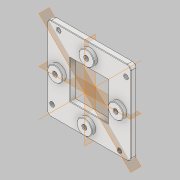
# Autodesk Inventor part: BaseTop
Saved by Autodesk Inventor 2019.2 (Build 232265000, 265)
## iProperties
Created: 2019-01-12
Part Number: BaseTop
Material: ABS-Kunststoff
Document SubType Name: Modeling
Designer: Lion
Density: 1.06 g/cm^3
Appearance: Weiß
Mass: 6.25719 g
Surface Area: 43.195 cm^2
Volume: 5.90301 cm^3
Author: Lion
## iProperties of the stored document BaseTop_3D-Druck.ipt
Created: 2019-04-11
Part Number: BaseTop_3D-Druck
Material: Generisch
Document SubType Name: Modeling
Designer: Lion
Density: 1 g/cm^3
Appearance: Vorgabe
Author: Lion
Autodesk Inventor part; units mm, degrees
ref_plane "YZ Plane" through (0, 0, 0) normal (1, 0, 0) x (0, 1, 0)
ref_plane "XZ Plane" through (0, 0, 0) normal (0, 1, 0) x (-1, 0, 0)
ref_plane "XY Plane" through (0, 0, 0) normal (0, 0, 1) x (1, 0, 0)
sketch "Skizze2" plane through (0, 0, 0) normal (0, 0, 1) x (1, 0, 0)
  line L0 (-16, -6) -> (16, -6)
  line L1 (16, -6) -> (16, 6)
  line L2 (16, 6) -> (-16, 6)
  line L3 (-16, 6) -> (-16, -6)
  line L4 (-16, -6) -> (16, 6) construction
  line L5 (16, -6) -> (-16, 6) construction
  line L6 (-11, 6) -> (3, 6)
  line L7 (3, 6) -> (3, -6)
  line L8 (3, -6) -> (-11, -6)
  line L9 (-11, -6) -> (-11, 6)
  circle A0 centre (-13.5, 0) radius 1
  line L10 (-11, -6) -> (-16, 6) construction
  line L11 (-16, -6) -> (-11, 6) construction
  line L12 (0, 6) -> (0, -6) construction
  circle A1 centre (13.5, 0) radius 1
  line L13 (-16, -21) -> (-28, -26) construction
  line L14 (-28, -7) -> (-16, -7)
  line L15 (-28, -10) -> (-16, -10) construction
  line L16 (-16, -26) -> (-16, 6)
  line L17 (-28, 6) -> (-28, -26)
  line L18 (-16, -26) -> (-28, 6) construction
  line L19 (-16, 6) -> (-28, -26) construction
  line L20 (-16, -21) -> (-28, -21)
  line L21 (-16, -7) -> (-16, -21)
  line L22 (-16, -26) -> (-28, -21) construction
  line L23 (-28, -26) -> (-16, -26)
  circle A2 centre (-22, -23.5) radius 1
  line L24 (-28, -21) -> (-28, -7)
  circle A3 centre (-22, 3.5) radius 1
  line L25 (-16, 6) -> (-28, 6)
  line L26 (-15, -38) -> (-15, -26)
  circle A4 centre (-25.5, -32) radius 1
  line L27 (-28, -26) -> (-28, -38)
  line L28 (-12, -38) -> (-12, -26) construction
  line L29 (4, -26) -> (-28, -26)
  line L30 (-28, -26) -> (4, -38) construction
  line L31 (4, -26) -> (-28, -38) construction
  line L32 (-28, -38) -> (4, -38)
  line L33 (-15, -26) -> (-1, -26)
  line L34 (-1, -38) -> (-15, -38)
  line L35 (-1, -26) -> (-1, -38)
  circle A5 centre (1.5, -32) radius 1
  line L36 (4, -26) -> (-1, -38) construction
  line L37 (-1, -26) -> (4, -38) construction
  line L38 (4, -38) -> (4, -26)
  line L39 (16, -25) -> (4, -25)
  circle A6 centre (10, -35.5) radius 1
  line L40 (4, -38) -> (16, -38)
  line L41 (16, -22) -> (4, -22) construction
  line L42 (4, -6) -> (4, -38)
  line L43 (4, -38) -> (16, -6) construction
  line L44 (4, -6) -> (16, -38) construction
  line L45 (16, -38) -> (16, -6)
  line L46 (4, -25) -> (4, -11)
  line L47 (16, -11) -> (16, -25)
  line L48 (4, -11) -> (16, -11)
  circle A7 centre (10, -8.5) radius 1
  line L49 (4, -6) -> (16, -11) construction
  line L50 (4, -11) -> (16, -6) construction
  line L51 (16, -6) -> (4, -6)
  line L52 (-16, -26) -> (4, -6) construction
  line L53 (4, -26) -> (-16, -6) construction
  line L54 (1, -23) -> (-13, -23)
  line L55 (-13, -23) -> (-13, -9)
  line L56 (-13, -9) -> (1, -9)
  line L57 (1, -9) -> (1, -23)
  line L58 (1, -23) -> (-13, -9) construction
  line L59 (-13, -23) -> (1, -9) construction
  line L60 (4, -25) -> (16, -25)
  line L61 (16, -25) -> (16, -38)
  line L62 (16, -38) -> (4, -38)
  line L63 (4, -38) -> (4, -25)
  point P0 (0, 0)
  point P1 (-13.5, 0)
  point P2 (-22, -10)
  point P3 (-12, -32)
  point P4 (10, -22)
  point P5 (-6, -16)
sketch "Skizze3" plane through (0, 0, 0) normal (0, 0, 1) x (1, 0, 0)
  circle A0 centre (-25.5, -32) radius 1 construction
  circle A1 centre (10, -35.5) radius 1 construction
  circle A2 centre (-22, 3.5) radius 1 construction
  circle A3 centre (13.5, 0) radius 1 construction
  line L0 (-28, 6) -> (16, 6)
  line L1 (16, 6) -> (16, -38)
  line L2 (16, -38) -> (-28, -38)
  line L3 (-28, -38) -> (-28, 6)
  circle A4 centre (-22, 3.5) radius 1
  circle A5 centre (13.5, 0) radius 1
  circle A6 centre (10, -35.5) radius 1
  circle A7 centre (-25.5, -32) radius 1
  line L4 (-16, -6) -> (4, -6)
  line L5 (4, -6) -> (4, -26)
  line L6 (4, -26) -> (-16, -26)
  line L7 (-16, -26) -> (-16, -6)
  line L8 (-11, -6) -> (-11, 6) construction
  line L9 (4, -11) -> (16, -11) construction
  line L10 (-1, -26) -> (-1, -38) construction
  line L11 (-16, -21) -> (-28, -21) construction
  circle A8 centre (-22, -15.5) radius 1.05
  line L12 (-22, -10) -> (-22, -23.5) construction
  line L13 (-12, -32) -> (1.5, -32) construction
  line L14 (10, -22) -> (10, -8.5) construction
  line L15 (-13.5, 0) -> (0, 0) construction
  circle A9 centre (10, -16.5) radius 1.05
  circle A10 centre (-5.5, 0) radius 1.05
  circle A11 centre (-6.5, -32) radius 1.05
  point P0 (-28, -38)
  point P1 (16, 6)
  point P2 (-16, -26)
  point P3 (4, -6)
  dimension "leghole_top_d" = 2.1
  dimension "d2" = 5.5
  dimension "d3" = 2.1
  dimension "d4" = 2.1
  dimension "d5" = 2.1
  dimension "d6" = 5.5
  dimension "d7" = 5.5
  dimension "d8" = 5.5
  constraints: 24 end point, 8 centre point, 4 coincident, 4 concentric, 4 horizontal, 4 parallel, 4 point on line, 2 perpendicular, 2 vertical
  measures "leghole_top_d" diameter of A8
  measures "d2" distance from line of L11 A8.centre
  measures "d3" diameter of A9
  measures "d4" diameter of A10
  measures "d5" diameter of A11
  measures "d6" distance from line of A11.centre L10
  measures "d7" distance from line of L9 A9.centre
  measures "d8" distance from line of L8 A10.centre
extrude "Extrusion1" add sketch "Skizze3" along normal blind 3
sketch "Skizze6" plane through (0, 0, 3) normal (0, 0, 1) x (1, 0, 0)
  circle A0 centre (-5.5, 0) radius 1.05 projected
  circle A1 centre (10, -16.5) radius 1.05 projected
  circle A2 centre (-22, -15.5) radius 1.05 projected
  circle A3 centre (-6.5, -32) radius 1.05 projected
  circle A4 centre (-5.5, 0) radius 4
  circle A5 centre (10, -16.5) radius 4
  circle A6 centre (-6.5, -32) radius 1.05 projected
  circle A7 centre (-6.5, -32) radius 4
  circle A8 centre (-22, -15.5) radius 4
  point P0 (0, 0)
  dimension "d18" = 8
  constraints: 4 centre point, 4 coincident, 3 equal radius
  measures "d18" diameter of A4
extrude "Extrusion3" add sketch "Skizze6" along normal blind 2
fillet "Rundung1" radius 2 4 edges at (-28, -38, 1.5) (16, -38, 1.5) (16, 6, 1.5) (-28, 6, 1.5)
ref_plane "Arbeitsebene1" through (-16, -6, 0) normal (0.7071068, 0.7071068, 0) x (0, 0, 1)
ref_plane "Arbeitsebene2" through (-16, -26, 0) normal (-0.7071068, 0.7071068, 0) x (0, 0, 1)
ref_plane "Arbeitsebene3" through (-6, -36, 0) normal (1, 0, 0) x (0, 0, -1)
ref_plane "Arbeitsebene4" through (-26, -16, 0) normal (0, 1, 0) x (1, 0, 0)
fillet "Rundung2" radius 0.25 44 edges at (-6, 6, 0) (-6, 6, 3) (-27.4142, 5.4142, 0) (15.4142, 5.4142, 0) (-28, -16, 0) (16, -16, 0) (-27.4142, -37.4142, 0) (15.4142, -37.4142, 0) (-6, -38, 0) (-26.5, -32, 0) (-7.55, -32, 0) (9, -35.5, 0) (8.95, -16.5, 0) (-23.05, -15.5, 0) (-16, -16, 0) (-6, -26, 0) (4, -16, 0) (-6, -6, 0) (-23, 3.5, 0) (-6.55, 0, 0) (12.5, 0, 0) (-27.4142, 5.4142, 3) (15.4142, 5.4142, 3) (-28, -16, 3) (16, -16, 3) (-27.4142, -37.4142, 3) (15.4142, -37.4142, 3) (-6, -38, 3) (-26.5, -32, 3) (9, -35.5, 3) (-16, -16, 3) (-6, -26, 3) (-6, -6, 3) (4, -16, 3) (-23, 3.5, 3) (12.5, 0, 3) (-7.55, -32, 5) (8.95, -16.5, 5) (-23.05, -15.5, 5) (-6.55, 0, 5) (-10.5, -32, 5) (6, -16.5, 5) (-26, -15.5, 5) (-9.5, 0, 5)
equation "\"d3\" = leghole_top_d"
equation "\"d4\" = leghole_top_d"
equation "\"d5\" = leghole_top_d"
